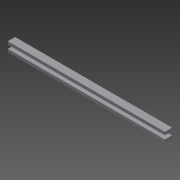
# Autodesk Inventor part: top_cover_end
Saved by Autodesk Inventor 2014 SP1 (Build 180222100, 222)
## iProperties
Created: 2014-02-23
Part Number: top_cover_end
Material: Generic
Document SubType Name: Modeling
Designer: Chris
Density: 1 g/cm^3
Appearance: Default
Mass: 158.814 g
Surface Area: 453.427 cm^2
Volume: 158.814 cm^3
Author: Chris
Autodesk Inventor part; units mm, degrees
ref_plane "YZ Plane" through (0, 0, 0) normal (1, 0, 0) x (0, 1, 0)
ref_plane "XZ Plane" through (0, 0, 0) normal (0, 1, 0) x (-1, 0, 0)
ref_plane "XY Plane" through (0, 0, 0) normal (0, 0, 1) x (1, 0, 0)
sketch "Sketch1" plane through (0, 0, 0) normal (0, 0, 1) x (1, 0, 0)
  line L0 (-277.5467, 56.2236) -> (135.2033, 56.2236)
  line L1 (-277.5467, 56.2236) -> (-277.5467, 48.2861)
  line L2 (-277.5467, 48.2861) -> (-258.4967, 48.2861)
  line L3 (-258.4967, 48.2861) -> (-258.4967, 38.7611)
  line L4 (-258.4967, 38.7611) -> (-277.5467, 38.7611)
  line L5 (-277.5467, 38.7611) -> (-277.5467, 30.8236)
  line L6 (-277.5467, 30.8236) -> (135.2033, 30.8236)
  line L7 (135.2033, 30.8236) -> (135.2033, 38.7611)
  line L8 (135.2033, 38.7611) -> (116.1533, 38.7611)
  line L9 (116.1533, 38.7611) -> (116.1533, 48.2861)
  line L10 (116.1533, 48.2861) -> (135.2033, 48.2861)
  line L11 (135.2033, 48.2861) -> (135.2033, 56.2236)
  point P0 (0, 0)
  dimension "d0" = 412.75
  dimension "d1" = 7.9375
  dimension "d2" = 7.9375
  dimension "d3" = 9.525
  dimension "d4" = 7.9375
  dimension "d5" = 9.525
  dimension "d6" = 19.05
  dimension "d7" = 19.05
  dimension "d8" = 19.05
  dimension "d14" = 412.75
  constraints: 24 end point, 6 parallel, 3 perpendicular, 2 collinear, 1 horizontal
  measures "d0" distance of L0.start L0.end
  measures "d1" distance of L0.start L1.end
  measures "d2" distance of L4.end L5.end
  measures "d3" distance of L2.end L3.end
  measures "d4" distance of L10.end L0.end
  measures "d5" distance of L8.end L9.end
  measures "d6" distance between parallel lines of L11 L9
  measures "d7" distance of L1.end L2.end
  measures "d8" distance of L3.end L4.end
  measures "d14" distance between parallel lines of L7 L5
extrude "Extrusion1" add sketch "Sketch1" along normal blind 19.05
sketch "Sketch2" plane through (0, 0, 19.05) normal (0, 0, 1) x (1, 0, 0)
  line L0 (-258.4967, 48.2861) -> (116.1533, 48.2861)
  line L1 (116.1533, 48.2861) -> (116.1533, 38.7611)
  line L2 (116.1533, 38.7611) -> (-258.4967, 38.7611)
  line L3 (-258.4967, 38.7611) -> (-258.4967, 48.2861)
  point P0 (0, 0)
  constraints: 8 end point, 2 parallel, 1 horizontal, 1 perpendicular
extrude "Extrusion2" cut sketch "Sketch2" against normal blind 9.525
equation "\"d14\" = d0"
body "Solid1"
